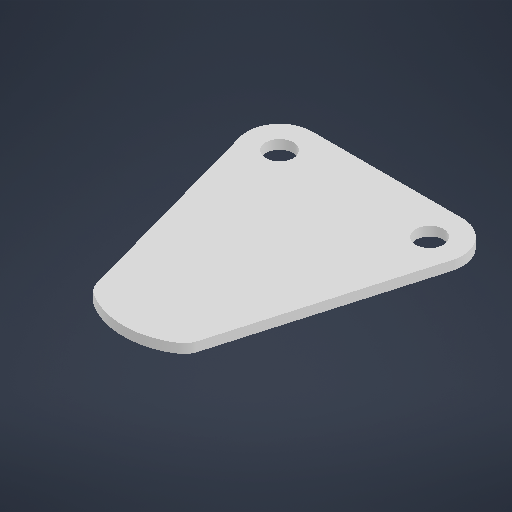
# Autodesk Inventor part: Hooks
Saved by Autodesk Inventor 2025.2 (Build 292293000, 293)
## iProperties
Created: 2025-01-26
Part Number: Hooks
Material: Generic
Document SubType Name: Sheet Metal
Designer: casey
Density: 1 g/cm^3
Appearance: Default
Flat Pattern Width: 3.54174 cm
Flat Pattern Length: 4.70281 cm
Flat Pattern Area: 16.6561 cm^2
Sheet Metal Rule: Default_mm
Sheet Metal Width: 1.394 in
Sheet Metal Length: 1.851 in
Sheet Metal Area: 2.582 in^2
Author: casey
Autodesk Inventor part; units mm, degrees
ref_plane "YZ Plane" through (0, 0, 0) normal (1, 0, 0) x (0, 1, 0)
ref_plane "XZ Plane" through (0, 0, 0) normal (0, 1, 0) x (-1, 0, 0)
ref_plane "XY Plane" through (0, 0, 0) normal (0, 0, 1) x (1, 0, 0)
sketch "Sketch1" plane through (0, 0, 0) normal (0, 1, 0) x (-1, 0, 0)
  arc A0 (-20.4896, -15.6558) -> (-14.6923, -22.2603) centre (-15.0688, -16.7442) ccw
  line L0 (-14.6923, -22.2603) -> (10.3315, -22.2603)
  arc A1 (-20.4896, -15.6558) -> (-14.6923, -22.2603) centre (-15.0688, -16.7442) ccw
  line L1 (-14.6923, -22.2603) -> (10.3315, -22.2603)
  line L2 (-14.6923, -22.2603) -> (10.3349, -22.2603)
  arc A2 (10.3349, -22.2603) -> (15.722, -15.6686) centre (10.3349, -16.7631) ccw
  line L3 (15.722, -15.6686) -> (6.3158, 18.2544)
  arc A3 (6.3158, 18.2544) -> (4.984, 20.0698) centre (3.2562, 17.406) ccw
  arc A4 (4.984, 20.0698) -> (-9.366, 20.0568) centre (-2.181, 9.023) ccw
  arc A5 (-9.366, 20.0568) -> (-10.6837, 18.2776) centre (-7.6335, 17.3962) ccw
  line L4 (-10.6837, 18.2776) -> (-20.4896, -15.6558)
  arc A6 (-20.4896, -15.6558) -> (-14.6923, -22.2603) centre (-15.0688, -16.7442) ccw
  line L5 (-14.6923, -22.2603) -> (10.3315, -22.2603)
  line L6 (-14.6923, -22.2603) -> (10.3315, -22.2603)
  circle A7 centre (10.3315, -16.7442) radius 2.3368
  circle A8 centre (10.3315, -16.7442) radius 2.3368
  circle A9 centre (10.3315, -16.7442) radius 2.3368
  circle A10 centre (10.3315, -16.7442) radius 2.3368
  circle A11 centre (-15.0688, -16.7442) radius 2.3368
  circle A12 centre (-15.0688, -16.7442) radius 2.3368
  circle A13 centre (-15.0688, -16.7442) radius 2.3368
  circle A14 centre (-15.0688, -16.7442) radius 2.3368
  circle A15 centre (-15.0688, -16.7442) radius 2.3368
  circle A16 centre (-15.0688, -16.7442) radius 2.3368
  line L7 (-14.6923, -22.2603) -> (10.3315, -22.2603)
  circle A17 centre (10.3315, -16.7442) radius 2.3368
  circle A18 centre (10.3315, -16.7442) radius 2.3368
  arc A19 (-20.4896, -15.6558) -> (-14.6923, -22.2603) centre (-15.0688, -16.7442) ccw
  arc A20 (-20.4896, -15.6558) -> (-14.6923, -22.2603) centre (-15.0688, -16.7442) ccw
  arc A21 (-20.4896, -15.6558) -> (-14.6923, -22.2603) centre (-15.0688, -16.7442) ccw
  point P0 (0, 0)
  point P1 (-10.6837, 18.2776)
  point P2 (-14.6923, -22.2603)
  point P3 (10.3349, -22.2603)
  point P4 (-9.366, 20.0568)
  constraints: 22 centre point, 20 point on circle, 16 end point
extrude "Extrusion1" add sketch "Sketch1" along normal blind 1.5875
equation "\"BendRadius\" = Thickness"
equation "\"BendReliefWidth\" = Thickness"
equation "\"BendReliefDepth\" = 0.5 * Thickness"
equation "\"CornerReliefSize\" = 4 * Thickness"
equation "\"MinimumRemnant\" = 2 * Thickness"
equation "\"TransitionRadius\" = BendRadius"
equation "\"JacobiRadiusSize\" = BendRadius"
equation "\"GapSize\" = Thickness"
equation "\"Thickness\" = 1.5875"
body "Solid1"
